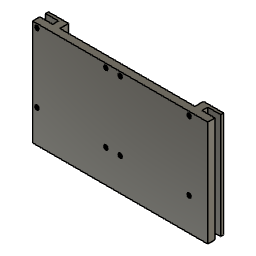
모터드라이버 브라켓 (Autodesk Fusion 360 design; units mm, degrees)
Autodesk Fusion 360 part; units mm, degrees
sketch "스케치1" plane through (0, 0, 0) normal (0, 1, 0) x (1, 0, 0)
  line L0 (-61, -36.75) -> (61, -36.75)
  line L1 (61, -36.75) -> (61, 36.75)
  line L2 (61, 36.75) -> (-61, 36.75)
  line L3 (-61, 36.75) -> (-61, -36.75)
  line L4 (-61, -36.75) -> (61, 36.75) construction
  line L5 (61, -36.75) -> (-61, 36.75) construction
  line L6 (61, 36.75) -> (-61, 36.75)
  line L7 (-61, 36.75) -> (-61, 16.75)
  line L8 (-61, 16.75) -> (61, 16.75)
  line L9 (61, 16.75) -> (61, 36.75)
  line L10 (-61, -36.75) -> (-61, -10)
  line L11 (-61, -10) -> (-34, -10)
  line L12 (-10, -34) -> (-58, -34)
  line L13 (-58, -34) -> (-58, 14)
  line L14 (-58, 14) -> (-10, 14)
  line L15 (-10, 14) -> (-10, -34)
  line L16 (-10, -34) -> (-58, 14) construction
  line L17 (-58, -34) -> (-10, 14) construction
  line L18 (-34, -10) -> (24, -10)
  line L19 (48, -34) -> (0, -34)
  line L20 (0, -34) -> (0, 14)
  line L21 (0, 14) -> (48, 14)
  line L22 (48, 14) -> (48, -34)
  line L23 (48, -34) -> (0, 14) construction
  line L24 (0, -34) -> (48, 14) construction
  circle A0 centre (-58, -34) radius 1.6
  circle A1 centre (-10, -34) radius 1.6
  circle A2 centre (-58, 14) radius 1.6
  circle A3 centre (-10, 14) radius 1.6
  circle A4 centre (0, -34) radius 1.6
  circle A5 centre (48, -34) radius 1.6
  circle A6 centre (0, 14) radius 1.6
  circle A7 centre (48, 14) radius 1.6
  point P0 (-34, -10)
  point P1 (24, -10)
  dimension "d1" = 122
  dimension "d2" = 73.5
  dimension "d3" = 20
  dimension "d4" = 26.75
  dimension "d5" = 27
  dimension "d6" = 48
  dimension "d7" = 48
  dimension "d8" = 58
  dimension "d9" = 48
  dimension "d10" = 48
  dimension "d11" = 3.2
  dimension "d12" = 3.2
  dimension "d13" = 3.2
  dimension "d14" = 3.2
  dimension "d15" = 3.2
  dimension "d16" = 3.2
  dimension "d17" = 3.2
  dimension "d18" = 3.2
  constraint horizontal L0
  constraint perpendicular L0 L1
  constraint parallel L0 L2
  constraint parallel L1 L3
  constraint coincident L4 origin
  constraint coincident L5 origin
  constraint horizontal L6
  constraint vertical L7
  constraint horizontal L8
  constraint vertical L9
  constraint coincident L3 L7.end
  constraint perpendicular L0 L10
  constraint perpendicular L3 L11
  constraint horizontal L12
  constraint perpendicular L12 L13
  constraint parallel L12 L14
  constraint parallel L13 L15
  constraint coincident L16 P0
  constraint coincident L17 P0
  constraint coincident P0 L11.end
  constraint perpendicular L15 L18
  constraint horizontal L19
  constraint perpendicular L19 L20
  constraint parallel L19 L21
  constraint parallel L20 L22
  constraint coincident L23 P1
  constraint coincident L24 P1
  constraint coincident P1 L18.end
  constraint coincident L12.end L13.start
  constraint coincident L12.start L15.end
  constraint coincident L13.end L14.start
  constraint coincident L14.end L15.start
  constraint coincident L19.end L20.start
  constraint coincident L19.start L22.end
  constraint coincident L20.end L21.start
  constraint coincident L21.end L22.start
  measures "d1" distance of L1.end L2.end
  measures "d2" distance of L0.end L1.end
  measures "d3" distance of L1.end L8.end
  measures "d4" distance of L0.start L10.end
  measures "d5" distance of L10.end P0
  measures "d6" distance of L13.end L14.end
  measures "d7" distance of L12.end L13.end
  measures "d8" distance of P0 P1
  measures "d9" distance of L20.end L21.end
  measures "d10" distance of L19.end L20.end
  measures "d11" diameter of A0
  measures "d12" diameter of A1
  measures "d13" diameter of A2
  measures "d14" diameter of A3
  measures "d15" diameter of A4
  measures "d16" diameter of A5
  measures "d17" diameter of A6
  measures "d18" diameter of A7
extrude "돌출1" add sketch "스케치1" along normal blind 5 contours L0 L1 L3 L8 L10 | L1 L2 L3 L6 L7 L8 L9 | L11 L13 L14 L15 L18 A2 A3 | L11 L12 L13 L15 L18 A0 A1 | L19 L20 L21 L22 A4 A5 A6 A7
sketch "스케치2" plane through (0, 5, 0) normal (0, 1, 0) x (-1, 0, 0)
  circle A0 centre (58, -14) radius 1.6
  circle A1 centre (-48, 34) radius 1.6
  circle A2 centre (58, 34) radius 1.6
  circle A3 centre (10, 34) radius 1.6
  circle A4 centre (0, -14) radius 1.6
  circle A5 centre (0, 34) radius 1.6
  circle A6 centre (10, -14) radius 1.6
  circle A7 centre (-48, -14) radius 1.6
  line L0 (-61, 36.75) -> (-61, -36.75)
  line L1 (-61, -36.75) -> (61, -36.75)
  line L2 (61, -36.75) -> (61, 36.75)
  line L3 (61, 36.75) -> (-61, 36.75)
  line L4 (-61, 36.75) -> (-52, 36.75)
  line L5 (-52, 36.75) -> (-47, 36.75)
  line L6 (-47, 36.75) -> (-47, -36.75)
  line L7 (-47, -36.75) -> (-52, -36.75)
  line L8 (-52, -36.75) -> (-52, 36.75)
  line L9 (61, 36.75) -> (52, 36.75)
  line L10 (52, 36.75) -> (47, 36.75)
  line L11 (47, 36.75) -> (47, -36.75)
  line L12 (47, -36.75) -> (52, -36.75)
  line L13 (52, -36.75) -> (52, 36.75)
  dimension "d21" = 9
  dimension "d22" = 5
  dimension "d23" = 9
  dimension "d24" = 5
  constraint coincident L0.start L3.end
  constraint perpendicular L0 L4
  constraint horizontal L5
  constraint vertical L6
  constraint horizontal L7
  constraint vertical L8
  constraint coincident L1 L6.end
  constraint coincident L2.end L3.start
  constraint perpendicular L2 L9
  constraint horizontal L10
  constraint vertical L11
  constraint horizontal L12
  constraint vertical L13
  constraint coincident L1 L11.end
  measures "d21" distance of L0.start L4.end
  measures "d22" distance of L4.end L5.end
  measures "d23" distance of L2.end L9.end
  measures "d24" distance of L9.end L10.end
extrude "돌출2" add sketch "스케치2" along normal blind 6 contours A1 L6 | A1 A7 L1 L3 L5 L6 L7 L8 | A7 L6 | L1 L3 L10 L11 L12 L13 picked at (-47.8667, 34) picked at (-47.8138, -14.2316)
sketch "스케치3" plane through (52, 0, 0) normal (1, 0, 0) x (0, 1, 0)
  line L0 (5, 36.75) -> (5, -36.75)
  line L1 (5, -36.75) -> (11, -36.75)
  line L2 (11, -36.75) -> (11, 36.75)
  line L3 (11, 36.75) -> (5, 36.75)
  line L4 (11, 36.75) -> (9, 36.75)
  line L5 (9, 36.75) -> (9, -36.75)
  line L6 (9, -36.75) -> (11, -36.75)
  line L7 (11, -36.75) -> (11, 36.75)
  dimension "d27" = 2
  constraint horizontal L4
  constraint vertical L5
  constraint horizontal L6
  constraint vertical L7
  constraint coincident L2.end L3.start
  measures "d27" distance of L2.end L4.end
extrude "돌출3" add sketch "스케치3" along normal blind 9 contours L1 L2 L3 L4 L5 L6 L7
sketch "스케치4" plane through (-52, 0, 0) normal (-1, 0, 0) x (0, -1, 0)
  line L0 (-5, -36.75) -> (-5, 36.75)
  line L1 (-5, 36.75) -> (-11, 36.75)
  line L2 (-11, 36.75) -> (-11, -36.75)
  line L3 (-11, -36.75) -> (-5, -36.75)
  line L4 (-11, 36.75) -> (-9, 36.75)
  line L5 (-9, 36.75) -> (-9, -36.75)
  line L6 (-9, -36.75) -> (-11, -36.75)
  line L7 (-11, -36.75) -> (-11, 36.75)
  dimension "d30" = 2
  constraint horizontal L4
  constraint vertical L5
  constraint horizontal L6
  constraint vertical L7
  constraint coincident L1.end L2.start
  measures "d30" distance of L1.end L4.end
extrude "돌출4" add sketch "스케치4" along normal blind 9 contours L1 L2 L3 L4 L5 L6 L7
thread "나사산1" "ISO Metric profile 3.0 M3x0.5 6H" major diameter 3.086 minor diameter 2.529 pitch 0.5 angle 60 modelled right hand crest width 0.1368 on face at (47.0644, 3.3333, 35.2979) crest through (49.2645, 0.125, 34) on face at (-11.3653, 1.6667, 33.1657) crest through (-8.7355, 0.125, 34) on face at (-1.2257, 3.3333, 32.9715) crest through (1.2645, 0.125, 34) on face at (1.592, 3.3333, -14.1593) crest through (1.2645, 0.125, -14) on face at (-8.408, 3.3333, -14.1593) crest through (-8.7355, 0.125, -14) on face at (-56.408, 3.3333, -14.1593) crest through (-56.7355, 0.125, -14) on face at (-57.7222, 1.6667, 32.4243) crest through (-56.7355, 0.125, 34) on face at (47.0644, 3.3333, -12.7021) crest through (49.2645, 0.125, -14)
